Autodesk Inventor part; units mm, degrees
(part 2 of 2)
extrude "Cut10" cut sketch "Sketch17" against normal blind 1.5875 contours A326 L237 A12 | A12 L237 L26 L238 A326 | L237 A327 L238 L26 | A16 A304 | A16 A304 L215 A305 L30 E0 L31 | L31 E0 L30 A305 L216 A304 | A302 L31 | L31 A302 L213 A303 L214 | A324 L235 L33 E3 L30 | L30 E3 L33 L235 L26 L236 A324 | A300 L31 | L31 A300 L211 A301 L212 | L26 L235 A325 L236 | A298 L209 A299 L32 E1 L31 | L31 E1 L32 A299 L210 A298 | L234 A322 L233 L33 | L33 L233 L26 L234 | L26 L233 A323 L234 | L232 A320 L231 L33 | L33 L231 L26 L232 | L26 L231 A321 L232 | A318 L229 A319 L230 L33 E2 L32 | L32 E2 L33 L230 A318 | A189 A17 | A17 A189 L100 A188 L99 | A32 A190 | A32 A190 L101 A191 L102 | A36 A168 | A36 A168 L79 A169 L80 | L217 A40 | A40 L217 A307 L218 A306 | A46 A158 | A46 A158 L69 A159 L70 | A179 A47 | A47 A179 L90 A178 L89 | A49 A176 | A49 A176 L87 A177 L88 | A52 A316 | A52 A316 L227 A317 L228 | L247 A337 L248 L37 | L37 L248 A336 L247 | A332 L243 A333 L43 | L43 A333 L244 A332 | A330 L241 A331 L45 | L45 A331 L242 A330 | A201 L112 A200 L51 | L51 A200 L111 A201 | A181 L92 A180 L51 | L51 A180 L91 A181 | A186 L97 A187 L52 | L52 A187 L98 A186 | A206 L117 A207 L52 | L52 A207 L118 A206 | L76 A164 L75 L54 | L54 L75 A165 L76 | L74 A162 L73 L54 | L54 L73 A163 L74 | A155 L66 A154 L65 | A157 L68 A156 L67 | A171 L82 A170 L81 | A173 L84 A172 L83 | A175 L86 A174 L85 | A183 L94 A182 L93 | A185 L96 A184 L95 | A193 L104 A192 L103 | A195 L106 A194 L105 | A197 L108 A196 L107 | A199 L110 A198 L109 | A203 L114 A202 L113 | A205 L116 A204 L115 | A209 L120 A208 L119 | A211 L122 A210 L121 | A213 L124 A212 L123 | A215 L126 A214 L125 | A217 L128 A216 L127 | A219 L130 A218 L129 | A223 L134 A222 L133 | A225 L136 A224 L135 | A229 L140 A228 L139 | A231 L142 A230 L141 | A233 L144 A232 L143 | A243 L154 A242 L153 | A245 L156 A244 L155 | A263 L174 A262 L173 | A265 L176 A264 L175 | A283 L194 A282 L193 | A285 L196 A284 L195 | A295 L206 A294 L205 | A297 L208 A296 L207 | A309 L220 A308 L219 | A315 L226 A314 L225 | A329 L240 A328 L239 | A335 L246 A334 L245 | A339 L250 A338 L249 | A341 L252 A340 L251 | A343 L254 A342 L253 | A345 L256 A344 L255 | A347 L258 A346 L257 | A349 L260 A348 L259 picked at (-131.7459, 207.6032) picked at (-196.6505, 253.8134) picked at (-543.7391, 156.9299) picked at (-592.9268, 96.0219) picked at (-644.9189, 158.8055) picked at (-186.8014, 207.4396) picked at (-644.9189, 357.4495) picked at (-543.7391, 359.3251) picked at (-592.9268, 420.2331) picked at (-148.9478, 418.9462)
equation "\"d17\" = Thickness"
equation "\"d65\" = Thickness"
equation "\"BendRadius\" = Thickness"
equation "\"BendReliefWidth\" = Thickness"
equation "\"BendReliefDepth\" = 0.5 * Thickness"
equation "\"CornerReliefSize\" = 4 * Thickness"
equation "\"MinimumRemnant\" = 2 * Thickness"
equation "\"TransitionRadius\" = BendRadius"
equation "\"JacobiRadiusSize\" = Thickness"
equation "\"GapSize\" = Thickness"
equation "\"d2\" = BendRadius"
equation "\"Thickness\" = 1.5875"
body "Solid1"
